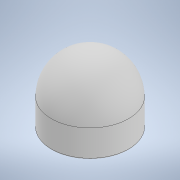
# Autodesk Inventor part: BlueYetiCap
Saved by Autodesk Inventor 2020 (Build 240168000, 168)
## iProperties
Created: 2020-07-23
Part Number: BlueYetiCap
Material: Generic
Document SubType Name: Modeling
Designer: maple
Density: 1 g/cm^3
Appearance: Default
Author: maple
Autodesk Inventor part; units mm, degrees
ref_plane "YZ Plane" through (0, 0, 0) normal (1, 0, 0) x (0, 1, 0)
ref_plane "XZ Plane" through (0, 0, 0) normal (0, 1, 0) x (-1, 0, 0)
ref_plane "XY Plane" through (0, 0, 0) normal (0, 0, 1) x (1, 0, 0)
sketch "Sketch1" plane through (0, 0, 0) normal (1, 0, 0) x (0, 1, 0)
  line L0 (0, 0) -> (-57, 0)
  line L1 (0, 0) -> (2, 0)
  line L2 (-57, 0) -> (-57, -32.5)
  line L3 (-57, -32.5) -> (-57, -34.5)
  line L4 (0, 0) -> (-32.5, 0)
  circle A0 centre (-32.5, 0) radius 32.5
  circle A1 centre (-32.5, 0) radius 34.5
  line L5 (-57, -32.5) -> (-32.5, -32.5)
  line L6 (-32.5, -34.5) -> (-57, -34.5)
  line L7 (0, 0) -> (2, 0)
  dimension "d0" = 57
  dimension "d1" = 2
  dimension "d2" = 32.5
  dimension "d3" = 2
  dimension "d4" = 32.5
  constraints: 16 end point, 4 horizontal, 4 point on circle, 2 centre point, 2 coincident, 2 point on line, 1 tangent, 1 vertical
  measures "d0" distance of L0.start L0.end
  measures "d1" distance of L0.start L1.end
  measures "d2" distance of L0.end L2.end
  measures "d3" distance of L2.end L3.end
  measures "d4" distance of L0.start L4.end
revolve "Revolution1" add sketch "Sketch1" angle 360 about axis through (0, 0, 0) along (0, -1, 0) contours L1 A1 L5 A0 | L6 L3 L5 A1
fillet "Fillet1" radius 1 1 edges at (0, -57, 34.5)
fillet "Fillet2" radius 1 1 edges at (0, -57, 32.5)
body "Solid1"
